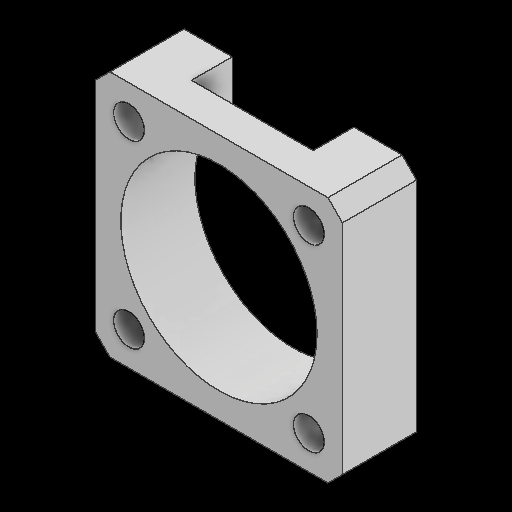
# Autodesk Inventor part: ArmEncoderSpacer
Saved by Autodesk Inventor 2025.2 (Build 292293000, 293)
## iProperties
Created: 2024-03-09
Part Number: ArmEncoderSpacer
Material: Generic
Document SubType Name: Modeling
Designer: valer
Density: 1 g/cm^3
Appearance: Default
Author: valer
Autodesk Inventor part; units mm, degrees
ref_plane "YZ Plane" through (0, 0, 0) normal (1, 0, 0) x (0, 1, 0)
ref_plane "XZ Plane" through (0, 0, 0) normal (0, 1, 0) x (-1, 0, 0)
ref_plane "XY Plane" through (0, 0, 0) normal (0, 0, 1) x (1, 0, 0)
sketch "Base" plane through (0, 0, 0) normal (0, 0, 1) x (1, 0, 0)
  line L0 (19.0001, -14.9999) -> (19.0001, 15.0001) projected
  line L1 (19.0001, 15.0001) -> (17.0001, 17.0001) projected
  line L2 (17.0001, 17.0001) -> (-12.9999, 17.0001) projected
  line L3 (-12.9999, 17.0001) -> (-14.9999, 15.0001) projected
  line L4 (-14.9999, 15.0001) -> (-14.9999, -14.9999) projected
  line L5 (-14.9999, -14.9999) -> (-12.9999, -16.9999) projected
  line L6 (-12.9999, -16.9999) -> (17.0001, -16.9999) projected
  line L7 (17.0001, -16.9999) -> (19.0001, -14.9999) projected
  circle A0 centre (-10.3744, 12.3746) radius 1.75 construction
  circle A1 centre (-2.9999, 8.7501) radius 0.475 construction
  circle A2 centre (-0.4999, 8.7501) radius 0.475 construction
  circle A3 centre (2.0001, 8.7501) radius 0.475 construction
  circle A4 centre (4.5001, 8.7501) radius 0.475 construction
  circle A5 centre (7.0001, 8.7501) radius 0.475 construction
  circle A6 centre (14.3746, 12.3746) radius 1.75 construction
  circle A7 centre (-10.3744, -12.3744) radius 1.75 construction
  circle A8 centre (14.3746, -12.3744) radius 1.75 construction
  line L8 (-5.7099, 9.0001) -> (-5.7099, 16.0001) construction
  line L9 (9.7101, 9.0001) -> (9.7101, 16.0001) construction
  line L10 (-5.7099, 16.0001) -> (9.7101, 16.0001) construction
  circle A9 centre (2, 0) radius 2.5 construction
  circle A10 centre (-10.3744, 12.3746) radius 4 construction
  circle A11 centre (14.3746, 12.3746) radius 4 construction
  circle A12 centre (14.3746, -12.3744) radius 4 construction
  circle A13 centre (-10.3744, -12.3744) radius 4 construction
  line L11 (-6.3744, 12.3746) -> (-6.3744, 17.0001)
  line L12 (10.3746, 12.3746) -> (10.3746, 17.0001)
  circle A14 centre (2, 0) radius 13.5002
  line L13 (-21.7999, 0) -> (25.8001, 0) construction
  line L14 (-6.3744, 12.3746) -> (-6.3744, 10.5889)
  line L15 (10.3746, 12.3746) -> (10.3746, 10.5887)
  circle A15 centre (-10.3744, 12.3746) radius 2.125
  circle A16 centre (-10.3744, -12.3744) radius 2.125
  circle A17 centre (14.3746, -12.3744) radius 2.125
  circle A18 centre (14.3746, 12.3746) radius 2.125
  point P0 (0, 0)
  point P1 (-7.5221, -9.57)
  point P2 (-7.57, -9.5221)
  dimension "d8" = 8
  dimension "d13" = 3.5
  dimension "d14" = 4.25
  constraints: 9 coincident, 8 end point, 7 centre point, 4 point on line, 3 equal radius, 2 horizontal alignment, 2 perpendicular, 2 point on circle, 2 vertical, 7 other
  measures "d13" diameter of A0
  measures "d14" diameter of A15
extrude "BaseFeature" add sketch "Base" along normal blind 10.2 contours L7 L6 L5 L4 L3 L2 L11 L14 A14 L15 L12 L1 L0 | L12 L15 A14 L14 L11 L2
extrude "ConnectorHoleFeature" cut sketch "Base" along normal blind 5.6 contours L12 L15 A14 L14 L11 L2
body "Solid2"
